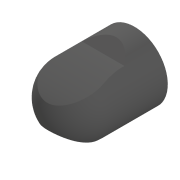
# Autodesk Inventor part: TipTip
Saved by Autodesk Inventor 2020 (Build 240168000, 168)
## iProperties
Created: 2021-03-25
Part Number: TipTip
Material: Generic
Document SubType Name: Modeling
Designer: deox
Density: 1 g/cm^3
Appearance: Generic
Author: deox
Autodesk Inventor part; units mm, degrees
ref_plane "YZ Plane" through (0, 0, 0) normal (1, 0, 0) x (0, 1, 0)
ref_plane "XZ Plane" through (0, 0, 0) normal (0, 1, 0) x (-1, 0, 0)
ref_plane "XY Plane" through (0, 0, 0) normal (0, 0, 1) x (1, 0, 0)
sketch "Sketch1" plane through (0, 0, 0) normal (0, 0, 1) x (1, 0, 0)
  circle A0 centre (0, 0) radius 6.75
  dimension "d0" = 13.5
  constraints: 1 centre point, 1 coincident
  measures "d0" diameter of A0
extrude "Extrusion1" add sketch "Sketch1" along normal blind 11.315
sketch "Sketch2" plane through (0, 0, 11.315) normal (0, 0, 1) x (1, 0, 0)
  arc A0 (0, -6.75) -> (0, 6.75) centre (0, 0) ccw
  line L0 (0, 6.75) -> (0, -6.75)
  constraints: 2 end point, 2 point on circle, 1 centre point, 1 coincident, 1 vertical
revolve "Revolution1" add sketch "Sketch2" angle 360 about axis through (0, 6.75, 11.315) along (0, -1, 0)
sketch "Sketch3" plane through (0, 0, 0) normal (1, 0, 0) x (0, 1, 0)
  line L0 (6.9939, 18.3652) -> (6.9939, -0.2867) construction
  line L1 (6.9939, -0.2867) -> (-6.6981, -0.2867) construction
  line L2 (-6.6981, -0.2867) -> (-6.6981, 18.3652) construction
  line L3 (-6.6981, 18.3652) -> (6.9939, 18.3652) construction
  line L4 (7.5187, 2.3916) -> (5.1843, 6.3459)
  spline S0 degree 3 poles (2.2232, 17.6743) (3.9137, 15.2739) (5.2905, 10.1216) (5.1843, 6.3459) knots 0 0 0 0 1 1 1 1
  spline S1 degree 4 poles (-2.7095, 17.5553) (-3.4345, 16.3323) (-3.9815, 15.3648) (-4.6404, 13.6169) (-5.2893, 11.6954) (-5.7416, 9.7633) (-6.0904, 7.9156) (-6.2555, 6.3812) (-6.4601, 3.9007) (-6.437, 2.3154) (-6.3311, 0.3242) (-6.2339, -0.1725) knots 0 0 0 0 0 0.226948 0.315631 0.407822 0.501079 0.595945 0.688744 0.781622 1 1 1 1 1
  arc A0 (2.2232, 17.6743) -> (-2.7095, 17.5553) centre (-0.2549, 18.1011) ccw
  line L5 (7.5187, 2.3916) -> (7.6074, -3.0566)
  line L6 (7.6074, -3.0566) -> (-6.5982, -2.034)
  line L7 (-6.5982, -2.034) -> (-6.1989, -0.3494)
  line L8 (-6.1989, -0.3494) -> (-6.2339, -0.1725)
  line L9 (-10.6943, 22.9274) -> (9.6594, 22.9274)
  line L10 (9.6594, 22.9274) -> (9.6594, -5.6031)
  line L11 (9.6594, -5.6031) -> (-10.6943, -5.6031)
  line L12 (-10.6943, -5.6031) -> (-10.6943, 22.9274)
  line L13 (-10.6943, 22.9274) -> (9.6594, -5.6031) construction
  line L14 (9.6594, 22.9274) -> (-10.6943, -5.6031) construction
  point P0 (0, 0)
  point P1 (3.606, 14.941)
  point P2 (4.8031, 10.6278)
  point P3 (-3.6969, 15.797)
  point P4 (-4.2759, 14.5167)
  point P5 (-4.7839, 13.1635)
  point P6 (-5.2449, 11.7299)
  point P7 (-5.7181, 9.7886)
  point P8 (-6.0639, 7.9039)
  point P9 (-6.252, 6.3205)
  point P10 (-6.3835, 4.5875)
  point P11 (-6.4199, 2.9071)
  point P12 (-6.3492, 0.98)
  point P13 (-0.5174, 8.6621)
  constraints: 22 end point, 2 midpoint, 2 parallel, 2 point on circle, 1 centre point, 1 horizontal, 1 perpendicular, 18 other
extrude "Extrusion2" cut sketch "Sketch3" against normal mid plane 15.315
sketch "Sketch4" plane through (0, 0, 0) normal (1, 0, 0) x (0, 1, 0)
  line L0 (0, 0) -> (4.875, 0)
  line L1 (6.75, 0) -> (-6.2616, 0) projected
  line L2 (4.875, 0) -> (4.875, 1.45)
  line L3 (4.875, 1.45) -> (5.56, 1.45)
  line L4 (5.56, 1.45) -> (5.56, 2.95)
  line L5 (5.56, 2.95) -> (5.56, 4.2347)
  line L6 (3.91, 4.3347) -> (5.56, 2.95)
  line L7 (0, 0) -> (0, 14.3)
  line L8 (0, 14.3) -> (3.1075, 14.3)
  line L9 (3.1075, 14.3) -> (3.91, 4.3347)
  dimension "d57" = 4.875
  dimension "d58" = 1.45
  dimension "d59" = 0.685
  dimension "d60" = 1.5
  dimension "d61" = 1.2847
  dimension "d63" = 14.3
  dimension "d64" = 3.1075
  constraints: 18 end point, 3 vertical, 2 perpendicular, 1 horizontal, 1 point on line
  measures "d57" distance of L0.start L0.end
  measures "d58" distance of L0.end L2.end
  measures "d59" distance of L2.end L3.end
  measures "d60" distance of L3.end L4.end
  measures "d61" distance of L4.end L5.end
  measures "d63" distance of L0.start L7.end
  measures "d64" distance of L7.end L8.end
revolve "Revolution2" cut sketch "Sketch4" angle 360 about axis through (0, 0, 0) along (0, 0, 1)
body "Solid1"
